Untitled_v4 (Autodesk Fusion 360 design; units mm, degrees)
Autodesk Fusion 360 part; units mm, degrees
(part 1 of 11)
sketch "Sketch1" plane through (0, 0, 0) normal (0, 1, 0) x (1, 0, 0)
  line L0 (0, -20) -> (0, 0)
  line L1 (0, 0) -> (20, 0)
  line L2 (20, 0) -> (0, -20)
  constraint coincident L0.end L1.start
  constraint vertical L0
  constraint perpendicular L0 L1
extrude "Extrude1" add sketch "Sketch1" along normal blind 220
extrude "Extrude2" add 1 faces at (6.6667, 73.3333, 0) along direction (0, 0, -1) blind 3
extrude "Extrude3" add 1 faces at (0, 73.3333, 12.3333) along direction (-1, 0, 0) blind 3
sketch "Sketch2" plane through (0, 0, -3) normal (0, 0, -1) x (1, 0, 0)
  line L0 (20, 0) -> (-3, 0)
  line L1 (-3, 0) -> (-3, -220)
  line L2 (-3, -220) -> (20, -220)
  line L3 (20, -220) -> (20, 0)
  line L4 (19.7694, -145.5685) -> (19.7946, -145.5378)
  line L5 (19.7422, -145.5975) -> (19.7694, -145.5685)
  line L6 (19.8738, -145.4005) -> (19.8878, -145.3633)
  line L7 (19.8177, -145.5055) -> (19.8387, -145.4717)
  line L8 (19.8878, -145.3633) -> (19.8993, -145.3253)
  line L9 (19.7946, -145.5378) -> (19.8177, -145.5055)
  line L10 (19.8574, -145.4367) -> (19.8738, -145.4005)
  line L11 (19.9083, -145.2866) -> (19.9148, -145.2474)
  line L12 (19.8574, -145.4367) -> (19.8738, -145.4005)
  line L13 (19.7946, -145.5378) -> (19.8177, -145.5055)
  line L14 (19.7422, -145.5975) -> (19.7694, -145.5685)
  line L15 (19.8738, -145.4005) -> (19.8878, -145.3633)
  arc A0 (19.92, -140.4997) -> (19.42, -139.9997) centre (19.42, -140.4997) ccw
  arc A1 (19.92, -140.4997) -> (19.42, -139.9997) centre (19.42, -140.4997) ccw
  line L16 (18.42, -139.9997) -> (19.42, -139.9997)
  line L17 (14.7514, -139.9997) -> (14.7117, -140.001)
  line L18 (14.7117, -139.9984) -> (14.7514, -139.9997)
  line L19 (14.7117, -139.9984) -> (14.7514, -139.9997)
  line L20 (14.7514, -139.9997) -> (14.7117, -140.001)
  arc A2 (19.42, -139.9997) -> (19.92, -139.4997) centre (19.42, -139.4997) ccw
  line L21 (18.42, -139.9997) -> (14.7514, -139.9997)
  line L22 (19.8993, -145.3253) -> (19.9083, -145.2866)
  line L23 (18.42, -139.9997) -> (14.7514, -139.9997)
  line L24 (18.42, -139.9997) -> (19.42, -139.9997)
  arc A3 (19.42, -139.9997) -> (19.92, -139.4997) centre (19.42, -139.4997) ccw
  line L25 (14.7514, -139.9997) -> (18.42, -139.9997)
  line L26 (14.7514, -139.9997) -> (18.42, -139.9997)
  line L27 (19.42, -139.9997) -> (18.42, -139.9997)
  line L28 (19.42, -139.9997) -> (18.42, -139.9997)
  line L29 (14.3819, -139.8742) -> (14.4142, -139.8974)
  line L30 (14.3222, -139.8219) -> (14.3512, -139.849)
  line L31 (14.5191, -140.0459) -> (14.483, -140.0623)
  line L32 (14.4142, -140.102) -> (14.3819, -140.1251)
  line L33 (14.483, -140.0623) -> (14.4479, -140.081)
  line L34 (14.3222, -139.8219) -> (14.3512, -139.849)
  line L35 (14.4479, -139.9183) -> (14.483, -139.9371)
  line L36 (14.3512, -140.1503) -> (14.3222, -140.1775)
  line L37 (14.3512, -139.849) -> (14.3819, -139.8742)
  line L38 (9.92, -146.3044) -> (9.7152, -146.0997)
  line L39 (14.483, -140.0623) -> (14.4479, -140.081)
  line L40 (14.3819, -139.8742) -> (14.4142, -139.8974)
  line L41 (14.483, -139.9371) -> (14.5191, -139.9534)
  line L42 (12.7593, -146.0997) -> (10.127, -146.0997)
  line L43 (14.3512, -139.849) -> (14.3819, -139.8742)
  line L44 (14.3819, -140.1251) -> (14.3512, -140.1503)
  line L45 (14.4142, -139.8974) -> (14.4479, -139.9183)
  line L46 (14.4479, -140.081) -> (14.4142, -140.102)
  line L47 (14.4479, -140.081) -> (14.4142, -140.102)
  line L48 (14.483, -139.9371) -> (14.5191, -139.9534)
  line L49 (14.3819, -140.1251) -> (14.3512, -140.1503)
  line L50 (14.4142, -139.8974) -> (14.4479, -139.9183)
  line L51 (14.4479, -139.9183) -> (14.483, -139.9371)
  line L52 (14.3512, -140.1503) -> (14.3222, -140.1775)
  line L53 (14.5191, -140.0459) -> (14.483, -140.0623)
  line L54 (14.4142, -140.102) -> (14.3819, -140.1251)
  line L55 (14.5943, -140.0203) -> (14.5563, -140.0319)
  line L56 (14.6722, -139.9945) -> (14.7117, -139.9984)
  line L57 (14.633, -139.988) -> (14.6722, -139.9945)
  line L58 (14.5943, -140.0203) -> (14.5563, -140.0319)
  line L59 (14.5563, -139.9674) -> (14.5943, -139.979)
  line L60 (14.6722, -140.0049) -> (14.633, -140.0113)
  line L61 (14.633, -140.0113) -> (14.5943, -140.0203)
  line L62 (14.6722, -139.9945) -> (14.7117, -139.9984)
  line L63 (14.633, -139.988) -> (14.6722, -139.9945)
  line L64 (14.6722, -140.0049) -> (14.633, -140.0113)
  line L65 (14.7117, -140.001) -> (14.6722, -140.0049)
  line L66 (14.5943, -139.979) -> (14.633, -139.988)
  line L67 (14.7117, -140.001) -> (14.6722, -140.0049)
  line L68 (14.5943, -139.979) -> (14.633, -139.988)
  line L69 (14.633, -140.0113) -> (14.5943, -140.0203)
  line L70 (14.5563, -139.9674) -> (14.5943, -139.979)
  line L71 (14.5563, -140.0319) -> (14.5191, -140.0459)
  line L72 (14.5191, -139.9534) -> (14.5563, -139.9674)
  line L73 (14.5563, -140.0319) -> (14.5191, -140.0459)
  line L74 (14.5191, -139.9534) -> (14.5563, -139.9674)
  line L75 (10.127, -146.0997) -> (9.92, -146.3044)
  line L76 (7.0807, -146.0997) -> (4.42, -143.439)
  line L77 (1.72, -144.4997) -> (3.3593, -144.4997)
  arc A4 (13.0414, -141.4582) -> (13.1828, -141.7997) centre (13.1828, -141.5997) ccw
  arc A5 (6.6572, -141.7997) -> (6.7986, -141.4582) centre (6.6572, -141.5997) ccw
  line L78 (9.92, -146.3044) -> (9.7152, -146.0997)
  line L79 (6.7986, -141.4582) -> (5.5178, -140.1775)
  line L80 (0.0978, -145.5975) -> (1.3786, -146.8782)
  line L81 (-0.08, -140.4997) -> (-0.08, -141.4997)
  line L82 (4.42, -143.439) -> (4.42, -141.7997)
  line L83 (4.42, -143.439) -> (4.42, -141.7997)
  line L84 (0.0978, -145.5975) -> (1.3786, -146.8782)
  line L85 (1.72, -144.4997) -> (3.3593, -144.4997)
  arc A6 (6.6572, -141.7997) -> (6.7986, -141.4582) centre (6.6572, -141.5997) ccw
  line L86 (7.0807, -146.0997) -> (4.42, -143.439)
  line L87 (4.42, -141.7997) -> (6.6572, -141.7997)
  line L88 (4.42, -141.7997) -> (6.6572, -141.7997)
  line L89 (-0.08, -140.4997) -> (-0.08, -141.4997)
  line L90 (6.7986, -141.4582) -> (5.5178, -140.1775)
  arc A7 (13.0414, -141.4582) -> (13.1828, -141.7997) centre (13.1828, -141.5997) ccw
  line L91 (12.7593, -146.0997) -> (10.127, -146.0997)
  line L92 (10.127, -146.0997) -> (9.92, -146.3044)
  line L93 (5.3209, -140.0459) -> (5.2837, -140.0319)
  line L94 (5.3209, -139.9534) -> (5.357, -139.9371)
  line L95 (5.357, -139.9371) -> (5.3921, -139.9183)
  line L96 (5.2837, -139.9674) -> (5.3209, -139.9534)
  line L97 (5.3209, -140.0459) -> (5.2837, -140.0319)
  line L98 (5.4888, -139.849) -> (5.5178, -139.8219)
  line L99 (5.4258, -140.102) -> (5.3921, -140.081)
  line L100 (5.0886, -139.9997) -> (5.1283, -139.9984)
  line L101 (5.3921, -140.081) -> (5.357, -140.0623)
  line L102 (5.3209, -139.9534) -> (5.357, -139.9371)
  line L103 (5.1283, -140.001) -> (5.0886, -139.9997)
  line L104 (5.0886, -139.9997) -> (5.1283, -139.9984)
  line L105 (5.1283, -140.001) -> (5.0886, -139.9997)
  line L106 (5.4581, -140.1251) -> (5.4258, -140.102)
  line L107 (5.4258, -139.8974) -> (5.4581, -139.8742)
  line L108 (5.2837, -139.9674) -> (5.3209, -139.9534)
  line L109 (5.3921, -139.9183) -> (5.4258, -139.8974)
  line L110 (5.357, -139.9371) -> (5.3921, -139.9183)
  line L111 (5.357, -140.0623) -> (5.3209, -140.0459)
  line L112 (5.4888, -140.1503) -> (5.4581, -140.1251)
  line L113 (5.3921, -139.9183) -> (5.4258, -139.8974)
  line L114 (5.4581, -140.1251) -> (5.4258, -140.102)
  line L115 (5.4258, -140.102) -> (5.3921, -140.081)
  line L116 (5.4258, -139.8974) -> (5.4581, -139.8742)
  line L117 (5.4581, -139.8742) -> (5.4888, -139.849)
  line L118 (5.3921, -140.081) -> (5.357, -140.0623)
  line L119 (5.357, -140.0623) -> (5.3209, -140.0459)
  line L120 (5.5178, -140.1775) -> (5.4888, -140.1503)
  line L121 (5.5178, -140.1775) -> (5.4888, -140.1503)
  line L122 (5.4888, -139.849) -> (5.5178, -139.8219)
  line L123 (-0.0174, -145.4367) -> (0.0013, -145.4717)
  line L124 (-0.0593, -145.3253) -> (-0.0478, -145.3633)
  line L125 (0.0706, -145.5685) -> (0.0978, -145.5975)
  line L126 (0.0454, -145.5378) -> (0.0706, -145.5685)
  line L127 (0.0454, -145.5378) -> (0.0706, -145.5685)
  line L128 (-0.0174, -145.4367) -> (0.0013, -145.4717)
  line L129 (-0.08, -141.4997) -> (-0.08, -145.0997)
  line L130 (-0.0683, -145.2866) -> (-0.0593, -145.3253)
  line L131 (-0.0593, -145.3253) -> (-0.0478, -145.3633)
  line L132 (-0.08, -145.0997) -> (-0.0787, -145.2079)
  line L133 (-0.0748, -145.2474) -> (-0.0683, -145.2866)
  line L134 (-0.0338, -145.4005) -> (-0.0174, -145.4367)
  line L135 (-0.0338, -145.4005) -> (-0.0174, -145.4367)
  line L136 (-0.0787, -145.2079) -> (-0.0748, -145.2474)
  line L137 (-0.0478, -145.3633) -> (-0.0338, -145.4005)
  line L138 (-0.08, -141.4997) -> (-0.08, -145.0997)
  line L139 (1.72, -146.7368) -> (1.72, -144.4997)
  line L140 (1.72, -146.7368) -> (1.72, -144.4997)
  line L141 (-0.0748, -145.2474) -> (-0.0683, -145.2866)
  line L142 (0.0706, -145.5685) -> (0.0978, -145.5975)
  line L143 (-0.0787, -145.2079) -> (-0.0748, -145.2474)
  line L144 (0.0223, -145.5055) -> (0.0454, -145.5378)
  line L145 (0.0013, -145.4717) -> (0.0223, -145.5055)
  line L146 (-0.08, -145.0997) -> (-0.0787, -145.2079)
  line L147 (0.0013, -145.4717) -> (0.0223, -145.5055)
  line L148 (-0.0478, -145.3633) -> (-0.0338, -145.4005)
  line L149 (0.0223, -145.5055) -> (0.0454, -145.5378)
  line L150 (-0.0683, -145.2866) -> (-0.0593, -145.3253)
  line L151 (18.12, -144.4997) -> (18.12, -146.7368)
  line L152 (16.4807, -144.4997) -> (18.12, -144.4997)
  line L153 (15.42, -141.7997) -> (15.42, -143.439)
  line L154 (15.42, -141.7997) -> (15.42, -143.439)
  line L155 (16.4807, -144.4997) -> (18.12, -144.4997)
  line L156 (18.12, -144.4997) -> (18.12, -146.7368)
  line L157 (5.207, -139.988) -> (5.2457, -139.979)
  line L158 (5.1283, -139.9984) -> (5.1678, -139.9945)
  line L159 (5.2457, -140.0203) -> (5.207, -140.0113)
  line L160 (5.1283, -139.9984) -> (5.1678, -139.9945)
  line L161 (5.2457, -139.979) -> (5.2837, -139.9674)
  line L162 (5.1678, -140.0049) -> (5.1283, -140.001)
  line L163 (5.2457, -140.0203) -> (5.207, -140.0113)
  line L164 (5.1678, -139.9945) -> (5.207, -139.988)
  line L165 (5.1678, -139.9945) -> (5.207, -139.988)
  line L166 (5.207, -140.0113) -> (5.1678, -140.0049)
  line L167 (5.207, -140.0113) -> (5.1678, -140.0049)
  line L168 (5.1678, -140.0049) -> (5.1283, -140.001)
  line L169 (5.207, -139.988) -> (5.2457, -139.979)
  line L170 (5.2837, -140.0319) -> (5.2457, -140.0203)
  line L171 (5.4581, -139.8742) -> (5.4888, -139.849)
  line L172 (5.4888, -140.1503) -> (5.4581, -140.1251)
  line L173 (5.2837, -140.0319) -> (5.2457, -140.0203)
  arc A8 (0.42, -139.9997) -> (-0.08, -140.4997) centre (0.42, -140.4997) ccw
  arc A9 (-0.08, -139.4997) -> (0.42, -139.9997) centre (0.42, -139.4997) ccw
  arc A10 (0.42, -139.9997) -> (-0.08, -140.4997) centre (0.42, -140.4997) ccw
  line L174 (1.42, -139.9997) -> (0.42, -139.9997)
  line L175 (5.0886, -139.9997) -> (1.42, -139.9997)
  line L176 (1.42, -139.9997) -> (5.0886, -139.9997)
  line L177 (0.42, -139.9997) -> (1.42, -139.9997)
  arc A11 (-0.08, -139.4997) -> (0.42, -139.9997) centre (0.42, -139.4997) ccw
  line L178 (0.42, -139.9997) -> (1.42, -139.9997)
  line L179 (1.42, -139.9997) -> (5.0886, -139.9997)
  line L180 (1.42, -139.9997) -> (0.42, -139.9997)
  line L181 (5.0886, -139.9997) -> (1.42, -139.9997)
  line L182 (5.2457, -139.979) -> (5.2837, -139.9674)
  line L183 (3.6807, -162.6997) -> (1.72, -162.6997)
  line L184 (7.0807, -166.0997) -> (3.6807, -162.6997)
  line L185 (0.0978, -165.5975) -> (1.3786, -166.8782)
  line L186 (3.6807, -162.6997) -> (1.72, -162.6997)
  line L187 (3.3593, -164.4997) -> (6.02, -167.1603)
  arc A12 (1.3786, -166.8782) -> (1.72, -166.7368) centre (1.52, -166.7368) ccw
  line L188 (1.72, -164.4997) -> (3.3593, -164.4997)
  arc A13 (1.3786, -166.8782) -> (1.72, -166.7368) centre (1.52, -166.7368) ccw
  line L189 (7.0807, -166.0997) -> (3.6807, -162.6997)
  line L190 (0.0978, -165.5975) -> (1.3786, -166.8782)
  line L191 (3.3593, -164.4997) -> (6.02, -167.1603)
  line L192 (1.72, -166.7368) -> (1.72, -164.4997)
  line L193 (1.72, -166.7368) -> (1.72, -164.4997)
  line L194 (1.72, -175.4997) -> (1.72, -173.2625)
  line L195 (-0.0593, -174.674) -> (-0.0683, -174.7127)
  line L196 (-0.0338, -174.5988) -> (-0.0478, -174.636)
  arc A14 (1.72, -173.2625) -> (1.3786, -173.1211) centre (1.52, -173.2625) ccw
  line L197 (0.0454, -174.4616) -> (0.0223, -174.4938)
  line L198 (-0.0174, -174.5626) -> (-0.0338, -174.5988)
  line L199 (0.0706, -174.4308) -> (0.0454, -174.4616)
  line L200 (1.72, -175.4997) -> (1.72, -173.2625)
  line L201 (0.0013, -174.5276) -> (-0.0174, -174.5626)
  line L202 (-0.0683, -174.7127) -> (-0.0748, -174.7519)
  line L203 (1.3786, -173.1211) -> (0.0978, -174.4019)
  line L204 (-0.0787, -174.7914) -> (-0.08, -174.8997)
  line L205 (0.0223, -174.4938) -> (0.0013, -174.5276)
  line L206 (-0.0787, -174.7914) -> (-0.08, -174.8997)
  line L207 (0.0454, -174.4616) -> (0.0223, -174.4938)
  line L208 (0.0013, -174.5276) -> (-0.0174, -174.5626)
  line L209 (-0.0748, -174.7519) -> (-0.0787, -174.7914)
  line L210 (0.0223, -174.4938) -> (0.0013, -174.5276)
  arc A15 (1.72, -173.2625) -> (1.3786, -173.1211) centre (1.52, -173.2625) ccw
  line L211 (-0.0683, -174.7127) -> (-0.0748, -174.7519)
  line L212 (0.0978, -174.4019) -> (0.0706, -174.4308)
  line L213 (0.0706, -174.4308) -> (0.0454, -174.4616)
  line L214 (0.0978, -174.4019) -> (0.0706, -174.4308)
  line L215 (-0.0174, -174.5626) -> (-0.0338, -174.5988)
  line L216 (1.3786, -173.1211) -> (0.0978, -174.4019)
  line L217 (-0.0748, -174.7519) -> (-0.0787, -174.7914)
  line L218 (-0.0338, -174.5988) -> (-0.0478, -174.636)
  line L219 (-0.0478, -174.636) -> (-0.0593, -174.674)
  line L220 (-0.0593, -174.674) -> (-0.0683, -174.7127)
  line L221 (-0.0478, -174.636) -> (-0.0593, -174.674)
  circle A16 centre (9.92, -109.9997) radius 2.1
  line L222 (6.02, -110.1995) -> (6.02, -112.839)
  line L223 (13.82, -112.839) -> (13.82, -110.1995)
  circle A17 centre (9.92, -109.9997) radius 2.1
  line L224 (-0.0174, -165.4367) -> (0.0013, -165.4717)
  line L225 (1.72, -164.4997) -> (3.3593, -164.4997)
  line L226 (-0.0683, -165.2866) -> (-0.0593, -165.3253)
  line L227 (0.0454, -165.5378) -> (0.0706, -165.5685)
  line L228 (0.0706, -165.5685) -> (0.0978, -165.5975)
  line L229 (0.0013, -165.4717) -> (0.0223, -165.5055)
  line L230 (0.0223, -165.5055) -> (0.0454, -165.5378)
  line L231 (-0.0748, -165.2474) -> (-0.0683, -165.2866)
  line L232 (-0.0338, -165.4005) -> (-0.0174, -165.4367)
  line L233 (0.0454, -165.5378) -> (0.0706, -165.5685)
  line L234 (-0.0478, -165.3633) -> (-0.0338, -165.4005)
  line L235 (-0.0338, -165.4005) -> (-0.0174, -165.4367)
  line L236 (0.0223, -165.5055) -> (0.0454, -165.5378)
  line L237 (3.3593, -124.4997) -> (6.02, -127.1603)
  line L238 (13.82, -127.1603) -> (16.4807, -124.4997)
  line L239 (5.5178, -139.8219) -> (6.7986, -138.5411)
  line L240 (13.82, -127.1603) -> (16.4807, -124.4997)
  line L241 (3.3593, -124.4997) -> (6.02, -127.1603)
  line L242 (5.5178, -139.8219) -> (6.7986, -138.5411)
  line L243 (13.0414, -138.5411) -> (14.3222, -139.8219)
  arc A18 (1.3786, -126.8782) -> (1.72, -126.7368) centre (1.52, -126.7368) ccw
  arc A19 (18.12, -126.7368) -> (18.4614, -126.8782) centre (18.32, -126.7368) ccw
  line L244 (13.0414, -138.5411) -> (14.3222, -139.8219)
  line L245 (19.92, -139.4997) -> (19.92, -138.4997)
  arc A20 (18.12, -126.7368) -> (18.4614, -126.8782) centre (18.32, -126.7368) ccw
  line L246 (19.92, -139.4997) -> (19.92, -138.4997)
  arc A21 (1.3786, -126.8782) -> (1.72, -126.7368) centre (1.52, -126.7368) ccw
  line L247 (-0.08, -138.4997) -> (-0.08, -139.4997)
  line L248 (-0.08, -138.4997) -> (-0.08, -139.4997)
  line L249 (0.0706, -165.5685) -> (0.0978, -165.5975)
  line L250 (-0.0787, -165.2079) -> (-0.0748, -165.2474)
  line L251 (-0.0748, -165.2474) -> (-0.0683, -165.2866)
  line L252 (-0.0683, -165.2866) -> (-0.0593, -165.3253)
  line L253 (-0.0174, -165.4367) -> (0.0013, -165.4717)
  line L254 (-0.08, -165.0997) -> (-0.0787, -165.2079)
  line L255 (0.0013, -165.4717) -> (0.0223, -165.5055)
  line L256 (-0.0593, -165.3253) -> (-0.0478, -165.3633)
  line L257 (-0.08, -165.0997) -> (-0.0787, -165.2079)
  line L258 (-0.0787, -165.2079) -> (-0.0748, -165.2474)
  line L259 (-0.0478, -165.3633) -> (-0.0338, -165.4005)
  line L260 (-0.0593, -165.3253) -> (-0.0478, -165.3633)
  line L261 (6.02, -112.839) -> (3.3593, -115.4997)
  line L262 (-0.08, -114.8997) -> (-0.08, -125.0997)
  line L263 (1.72, -122.6997) -> (1.72, -117.2997)
  line L264 (10.127, -126.0997) -> (9.92, -126.3066)
  line L265 (12.7593, -126.0997) -> (10.127, -126.0997)
  line L266 (-0.08, -114.8997) -> (-0.08, -125.0997)
  line L267 (1.72, -122.6997) -> (1.72, -117.2997)
  line L268 (-0.0787, -114.7914) -> (-0.08, -114.8997)
  line L269 (1.72, -117.2997) -> (3.6807, -117.2997)
  line L270 (3.3593, -115.4997) -> (1.72, -115.4997)
  line L271 (-0.0683, -114.7127) -> (-0.0748, -114.7519)
  line L272 (-0.0478, -114.636) -> (-0.0593, -114.674)
  line L273 (0.0454, -114.4616) -> (0.0223, -114.4938)
  line L274 (-0.0748, -114.7519) -> (-0.0787, -114.7914)
  line L275 (0.0706, -114.4308) -> (0.0454, -114.4616)
  line L276 (1.72, -115.4997) -> (1.72, -113.2625)
  line L277 (-0.0338, -114.5988) -> (-0.0478, -114.636)
  line L278 (0.0223, -114.4938) -> (0.0013, -114.5276)
  line L279 (-0.0174, -114.5626) -> (-0.0338, -114.5988)
  line L280 (6.02, -112.839) -> (3.3593, -115.4997)
  line L281 (1.72, -115.4997) -> (1.72, -113.2625)
  line L282 (-0.0174, -114.5626) -> (-0.0338, -114.5988)
  line L283 (-0.0683, -114.7127) -> (-0.0748, -114.7519)
  line L284 (0.0978, -114.4019) -> (0.0706, -114.4308)
  line L285 (0.0013, -114.5276) -> (-0.0174, -114.5626)
  line L286 (-0.0593, -114.674) -> (-0.0683, -114.7127)
  line L287 (3.3593, -115.4997) -> (1.72, -115.4997)
  line L288 (0.0013, -114.5276) -> (-0.0174, -114.5626)
  line L289 (0.0978, -114.4019) -> (0.0706, -114.4308)
  line L290 (1.3786, -113.1211) -> (0.0978, -114.4019)
  line L291 (-0.0787, -114.7914) -> (-0.08, -114.8997)
  line L292 (0.0706, -114.4308) -> (0.0454, -114.4616)
  line L293 (1.72, -117.2997) -> (3.6807, -117.2997)
  line L294 (-0.0338, -114.5988) -> (-0.0478, -114.636)
  arc A22 (1.72, -113.2625) -> (1.3786, -113.1211) centre (1.52, -113.2625) ccw
  line L295 (-0.0478, -114.636) -> (-0.0593, -114.674)
  line L296 (0.0454, -114.4616) -> (0.0223, -114.4938)
  arc A23 (1.72, -113.2625) -> (1.3786, -113.1211) centre (1.52, -113.2625) ccw
  line L297 (1.3786, -113.1211) -> (0.0978, -114.4019)
  line L298 (-0.0748, -114.7519) -> (-0.0787, -114.7914)
  line L299 (-0.0593, -114.674) -> (-0.0683, -114.7127)
  line L300 (0.0223, -114.4938) -> (0.0013, -114.5276)
  line L301 (0.0223, -134.4938) -> (0.0013, -134.5276)
  line L302 (0.0013, -134.5276) -> (-0.0174, -134.5626)
  line L303 (-0.0683, -134.7127) -> (-0.0748, -134.7519)
  line L304 (-0.08, -134.8997) -> (-0.08, -138.4997)
  line L305 (0.0978, -134.4019) -> (0.0706, -134.4308)
  line L306 (-0.0338, -134.5988) -> (-0.0478, -134.636)
  line L307 (0.0223, -134.4938) -> (0.0013, -134.5276)
  line L308 (0.0013, -134.5276) -> (-0.0174, -134.5626)
  line L309 (-0.0748, -134.7519) -> (-0.0787, -134.7914)
  line L310 (-0.0478, -134.636) -> (-0.0593, -134.674)
  line L311 (0.0978, -134.4019) -> (0.0706, -134.4308)
  line L312 (-0.0174, -134.5626) -> (-0.0338, -134.5988)
  line L313 (-0.0787, -134.7914) -> (-0.08, -134.8997)
  line L314 (0.0706, -134.4308) -> (0.0454, -134.4616)
  line L315 (6.6572, -138.1997) -> (4.42, -138.1997)
  line L316 (6.02, -129.7998) -> (6.2199, -129.9997)
  arc A24 (6.7986, -138.5411) -> (6.6572, -138.1997) centre (6.6572, -138.3997) ccw
  line L317 (4.42, -138.1997) -> (4.42, -136.5603)
  line L318 (6.02, -129.7998) -> (6.2199, -129.9997)
  arc A25 (6.7986, -138.5411) -> (6.6572, -138.1997) centre (6.6572, -138.3997) ccw
  line L319 (3.3593, -135.4997) -> (1.72, -135.4997)
  line L320 (3.3593, -135.4997) -> (1.72, -135.4997)
  line L321 (4.42, -138.1997) -> (4.42, -136.5603)
  line L322 (6.6572, -138.1997) -> (4.42, -138.1997)
  line L323 (6.02, -130.1995) -> (6.02, -132.839)
  arc A26 (1.72, -133.2625) -> (1.3786, -133.1211) centre (1.52, -133.2625) ccw
  line L324 (4.42, -136.5603) -> (7.0807, -133.8997)
  line L325 (6.02, -127.1603) -> (6.02, -129.7998)
  line L326 (6.2199, -129.9997) -> (6.02, -130.1995)
  line L327 (6.02, -132.839) -> (3.3593, -135.4997)
  line L328 (1.3786, -133.1211) -> (0.0978, -134.4019)
  line L329 (1.3786, -133.1211) -> (0.0978, -134.4019)
  line L330 (1.72, -135.4997) -> (1.72, -133.2625)
  arc A27 (1.72, -133.2625) -> (1.3786, -133.1211) centre (1.52, -133.2625) ccw
  line L331 (4.42, -136.5603) -> (7.0807, -133.8997)
  line L332 (6.02, -127.1603) -> (6.02, -129.7998)
  line L333 (6.2199, -129.9997) -> (6.02, -130.1995)
  line L334 (6.02, -130.1995) -> (6.02, -132.839)
  line L335 (6.02, -132.839) -> (3.3593, -135.4997)
  line L336 (1.72, -135.4997) -> (1.72, -133.2625)
  line L337 (13.6201, -129.9997) -> (13.82, -129.7998)
  line L338 (13.82, -132.839) -> (13.82, -130.1995)
  line L339 (9.92, -133.6949) -> (10.127, -133.8997)
  arc A28 (13.1828, -138.1997) -> (13.0414, -138.5411) centre (13.1828, -138.3997) ccw
  line L340 (9.7152, -133.8997) -> (9.92, -133.6949)
  line L341 (13.82, -129.7998) -> (13.82, -127.1603)
  line L342 (15.42, -136.5603) -> (15.42, -138.1997)
  line L343 (13.82, -129.7998) -> (13.82, -127.1603)
  line L344 (13.82, -130.1995) -> (13.6201, -129.9997)
  line L345 (19.7946, -134.4616) -> (19.7694, -134.4308)
  line L346 (19.92, -138.4997) -> (19.92, -134.8311)
  line L347 (16.4807, -135.4997) -> (13.82, -132.839)
  line L348 (18.12, -135.4997) -> (16.4807, -135.4997)
  circle A29 centre (9.92, -129.9997) radius 2.1
  circle A30 centre (9.92, -129.9997) radius 2.1
  line L349 (7.0807, -133.8997) -> (9.7152, -133.8997)
  line L350 (16.4807, -135.4997) -> (13.82, -132.839)
  line L351 (7.0807, -133.8997) -> (9.7152, -133.8997)
  line L352 (19.8878, -134.636) -> (19.8738, -134.5988)
  line L353 (-0.0174, -125.4367) -> (0.0013, -125.4717)
  line L354 (1.72, -124.4997) -> (3.3593, -124.4997)
  line L355 (0.0013, -125.4717) -> (0.0223, -125.5055)
  line L356 (-0.0683, -125.2866) -> (-0.0593, -125.3253)
  line L357 (-0.08, -125.0997) -> (-0.0787, -125.2079)
  line L358 (0.0706, -125.5685) -> (0.0978, -125.5975)
  line L359 (-0.08, -125.0997) -> (-0.0787, -125.2079)
  line L360 (-0.0478, -125.3633) -> (-0.0338, -125.4005)
  line L361 (-0.0338, -125.4005) -> (-0.0174, -125.4367)
  line L362 (-0.0593, -125.3253) -> (-0.0478, -125.3633)
  line L363 (1.72, -124.4997) -> (3.3593, -124.4997)
  line L364 (-0.0338, -125.4005) -> (-0.0174, -125.4367)
  line L365 (0.0223, -125.5055) -> (0.0454, -125.5378)
  line L366 (-0.0478, -125.3633) -> (-0.0338, -125.4005)
  line L367 (-0.0593, -125.3253) -> (-0.0478, -125.3633)
  line L368 (0.0978, -125.5975) -> (1.3786, -126.8782)
  line L369 (-0.0748, -125.2474) -> (-0.0683, -125.2866)
  line L370 (-0.0748, -125.2474) -> (-0.0683, -125.2866)
  line L371 (-0.0683, -125.2866) -> (-0.0593, -125.3253)
  line L372 (0.0454, -125.5378) -> (0.0706, -125.5685)
  line L373 (0.0223, -125.5055) -> (0.0454, -125.5378)
  line L374 (1.72, -126.7368) -> (1.72, -124.4997)
  line L375 (1.72, -126.7368) -> (1.72, -124.4997)
  line L376 (0.0706, -125.5685) -> (0.0978, -125.5975)
  line L377 (0.0013, -125.4717) -> (0.0223, -125.5055)
  line L378 (3.6807, -122.6997) -> (1.72, -122.6997)
  line L379 (-0.0787, -125.2079) -> (-0.0748, -125.2474)
  line L380 (-0.0174, -125.4367) -> (0.0013, -125.4717)
  line L381 (3.6807, -122.6997) -> (1.72, -122.6997)
  line L382 (0.0978, -125.5975) -> (1.3786, -126.8782)
  line L383 (0.0454, -125.5378) -> (0.0706, -125.5685)
  line L384 (-0.0787, -125.2079) -> (-0.0748, -125.2474)
  line L385 (19.8574, -134.5626) -> (19.8387, -134.5276)
  line L386 (19.9187, -134.7914) -> (19.9148, -134.7519)
  line L387 (19.7422, -134.4019) -> (18.4614, -133.1211)
  line L388 (19.8878, -134.636) -> (19.8738, -134.5988)
  line L389 (19.8574, -134.5626) -> (19.8387, -134.5276)
  line L390 (19.9083, -134.7127) -> (19.8993, -134.674)
  line L391 (19.92, -138.4997) -> (19.92, -134.8311)
  line L392 (19.8387, -134.5276) -> (19.8177, -134.4938)
  line L393 (19.9148, -134.7519) -> (19.9083, -134.7127)
  line L394 (19.8177, -134.4938) -> (19.7946, -134.4616)
  line L395 (19.8993, -134.674) -> (19.8878, -134.636)
  line L396 (19.9148, -134.7519) -> (19.9083, -134.7127)
  line L397 (19.7946, -134.4616) -> (19.7694, -134.4308)
  line L398 (19.7694, -134.4308) -> (19.7422, -134.4019)
  line L399 (19.8177, -134.4938) -> (19.7946, -134.4616)
  line L400 (19.9187, -134.7914) -> (19.9148, -134.7519)
  line L401 (12.7593, -133.8997) -> (15.42, -136.5603)
  line L402 (15.42, -138.1997) -> (13.1828, -138.1997)
  line L403 (13.6201, -129.9997) -> (13.82, -129.7998)
  line L404 (10.127, -133.8997) -> (12.7593, -133.8997)
  line L405 (13.82, -130.1995) -> (13.6201, -129.9997)
  line L406 (15.42, -136.5603) -> (15.42, -138.1997)
  line L407 (13.82, -132.839) -> (13.82, -130.1995)
  line L408 (10.127, -133.8997) -> (12.7593, -133.8997)
  line L409 (9.92, -133.6949) -> (10.127, -133.8997)
  line L410 (12.7593, -133.8997) -> (15.42, -136.5603)
  line L411 (15.42, -138.1997) -> (13.1828, -138.1997)
  line L412 (9.7152, -133.8997) -> (9.92, -133.6949)
  arc A31 (13.1828, -138.1997) -> (13.0414, -138.5411) centre (13.1828, -138.3997) ccw
  line L413 (19.8387, -134.5276) -> (19.8177, -134.4938)
  line L414 (18.12, -133.2625) -> (18.12, -135.4997)
  line L415 (18.12, -133.2625) -> (18.12, -135.4997)
  line L416 (19.7694, -134.4308) -> (19.7422, -134.4019)
  arc A32 (18.4614, -133.1211) -> (18.12, -133.2625) centre (18.32, -133.2625) ccw
  line L417 (18.12, -135.4997) -> (16.4807, -135.4997)
  line L418 (19.8738, -134.5988) -> (19.8574, -134.5626)
  line L419 (19.8993, -134.674) -> (19.8878, -134.636)
  line L420 (19.92, -134.8311) -> (19.9187, -134.7914)
  line L421 (19.7422, -134.4019) -> (18.4614, -133.1211)
  arc A33 (18.4614, -133.1211) -> (18.12, -133.2625) centre (18.32, -133.2625) ccw
  line L422 (19.9083, -134.7127) -> (19.8993, -134.674)
  line L423 (19.92, -134.8311) -> (19.9187, -134.7914)
  line L424 (19.8738, -134.5988) -> (19.8574, -134.5626)
  line L425 (19.92, -125.0997) -> (19.92, -114.8997)
  line L426 (16.1593, -122.6997) -> (12.7593, -126.0997)
  line L427 (3.6807, -117.2997) -> (7.0807, -113.8997)
  line L428 (19.92, -125.0997) -> (19.92, -114.8997)
  line L429 (19.8993, -114.674) -> (19.8878, -114.636)
  line L430 (18.12, -113.2625) -> (18.12, -115.4997)
  line L431 (16.1593, -122.6997) -> (12.7593, -126.0997)
  line L432 (19.8177, -114.4938) -> (19.7946, -114.4616)
  line L433 (16.4807, -115.4997) -> (13.82, -112.839)
  line L434 (18.12, -115.4997) -> (16.4807, -115.4997)
  line L435 (16.4807, -115.4997) -> (13.82, -112.839)
  line L436 (12.7593, -113.8997) -> (16.1593, -117.2997)
  line L437 (7.0807, -126.0997) -> (3.6807, -122.6997)
  line L438 (12.7593, -113.8997) -> (16.1593, -117.2997)
  line L439 (7.0807, -126.0997) -> (3.6807, -122.6997)
  line L440 (3.6807, -117.2997) -> (7.0807, -113.8997)
  line L441 (19.8993, -114.674) -> (19.8878, -114.636)
  line L442 (19.9083, -114.7127) -> (19.8993, -114.674)
  line L443 (19.8878, -114.636) -> (19.8738, -114.5988)
  arc A34 (18.4614, -113.1211) -> (18.12, -113.2625) centre (18.32, -113.2625) ccw
  line L444 (18.12, -122.6997) -> (16.1593, -122.6997)
  line L445 (19.8738, -114.5988) -> (19.8574, -114.5626)
  line L446 (19.8738, -114.5988) -> (19.8574, -114.5626)
  line L447 (19.7422, -114.4019) -> (18.4614, -113.1211)
  line L448 (18.12, -122.6997) -> (16.1593, -122.6997)
  line L449 (16.1593, -117.2997) -> (18.12, -117.2997)
  line L450 (19.7694, -114.4308) -> (19.7422, -114.4019)
  line L451 (19.92, -114.8997) -> (19.9187, -114.7914)
  line L452 (19.8387, -114.5276) -> (19.8177, -114.4938)
  line L453 (19.92, -114.8997) -> (19.9187, -114.7914)
  line L454 (19.9083, -114.7127) -> (19.8993, -114.674)
  line L455 (19.7946, -114.4616) -> (19.7694, -114.4308)
  line L456 (19.7422, -114.4019) -> (18.4614, -113.1211)
  line L457 (19.8878, -114.636) -> (19.8738, -114.5988)
  line L458 (18.12, -117.2997) -> (18.12, -122.6997)
  line L459 (19.9148, -114.7519) -> (19.9083, -114.7127)
  line L460 (19.8177, -114.4938) -> (19.7946, -114.4616)
  line L461 (16.1593, -117.2997) -> (18.12, -117.2997)
  line L462 (19.9187, -114.7914) -> (19.9148, -114.7519)
  line L463 (19.8574, -114.5626) -> (19.8387, -114.5276)
  line L464 (19.7946, -114.4616) -> (19.7694, -114.4308)
  line L465 (18.12, -117.2997) -> (18.12, -122.6997)
  line L466 (18.12, -115.4997) -> (16.4807, -115.4997)
  arc A35 (18.4614, -113.1211) -> (18.12, -113.2625) centre (18.32, -113.2625) ccw
  line L467 (19.9148, -114.7519) -> (19.9083, -114.7127)
  line L468 (19.7694, -114.4308) -> (19.7422, -114.4019)
  line L469 (19.9187, -114.7914) -> (19.9148, -114.7519)
  line L470 (19.8574, -114.5626) -> (19.8387, -114.5276)
  line L471 (19.8387, -114.5276) -> (19.8177, -114.4938)
  line L472 (18.12, -113.2625) -> (18.12, -115.4997)
  line L473 (19.9187, -125.2079) -> (19.92, -125.0997)
  line L474 (19.8878, -125.3633) -> (19.8993, -125.3253)
  line L475 (16.4807, -124.4997) -> (18.12, -124.4997)
  line L476 (19.7946, -125.5378) -> (19.8177, -125.5055)
  line L477 (19.9083, -125.2866) -> (19.9148, -125.2474)
  line L478 (19.9187, -125.2079) -> (19.92, -125.0997)
  line L479 (19.8177, -125.5055) -> (19.8387, -125.4717)
  line L480 (19.9148, -125.2474) -> (19.9187, -125.2079)
  line L481 (19.8177, -125.5055) -> (19.8387, -125.4717)
  line L482 (19.7694, -125.5685) -> (19.7946, -125.5378)
  line L483 (12.7593, -126.0997) -> (10.127, -126.0997)
  line L484 (9.92, -126.3066) -> (9.713, -126.0997)
  line L485 (9.92, -113.6927) -> (10.127, -113.8997)
  line L486 (10.127, -126.0997) -> (9.92, -126.3066)
  line L487 (9.92, -113.6927) -> (10.127, -113.8997)
  line L488 (10.127, -113.8997) -> (12.7593, -113.8997)
  line L489 (7.0807, -113.8997) -> (9.713, -113.8997)
  line L490 (9.713, -126.0997) -> (7.0807, -126.0997)
  line L491 (9.713, -113.8997) -> (9.92, -113.6927)
  line L492 (7.0807, -113.8997) -> (9.713, -113.8997)
  line L493 (9.713, -126.0997) -> (7.0807, -126.0997)
  line L494 (9.92, -126.3066) -> (9.713, -126.0997)
  line L495 (9.713, -113.8997) -> (9.92, -113.6927)
  line L496 (10.127, -113.8997) -> (12.7593, -113.8997)
  line L497 (18.12, -124.4997) -> (18.12, -126.7368)
  line L498 (19.8993, -125.3253) -> (19.9083, -125.2866)
  line L499 (19.7946, -125.5378) -> (19.8177, -125.5055)
  line L500 (19.8574, -125.4367) -> (19.8738, -125.4005)
  line L501 (19.7694, -125.5685) -> (19.7946, -125.5378)
  line L502 (19.7422, -125.5975) -> (19.7694, -125.5685)
  line L503 (19.8738, -125.4005) -> (19.8878, -125.3633)
  line L504 (18.4614, -126.8782) -> (19.7422, -125.5975)
  line L505 (19.8738, -125.4005) -> (19.8878, -125.3633)
  line L506 (19.8387, -125.4717) -> (19.8574, -125.4367)
  line L507 (19.8993, -125.3253) -> (19.9083, -125.2866)
  line L508 (19.7422, -125.5975) -> (19.7694, -125.5685)
  line L509 (16.4807, -124.4997) -> (18.12, -124.4997)
  line L510 (19.8387, -125.4717) -> (19.8574, -125.4367)
  line L511 (19.8878, -125.3633) -> (19.8993, -125.3253)
  line L512 (19.8574, -125.4367) -> (19.8738, -125.4005)
  line L513 (19.9083, -125.2866) -> (19.9148, -125.2474)
  line L514 (18.12, -124.4997) -> (18.12, -126.7368)
  line L515 (19.9148, -125.2474) -> (19.9187, -125.2079)
  line L516 (18.4614, -126.8782) -> (19.7422, -125.5975)
  line L517 (18.12, -153.2625) -> (18.12, -155.4997)
  line L518 (19.9083, -154.7127) -> (19.8993, -154.674)
  line L519 (19.9148, -154.7519) -> (19.9083, -154.7127)
  line L520 (19.9187, -154.7914) -> (19.9148, -154.7519)
  line L521 (19.8574, -154.5626) -> (19.8387, -154.5276)
  line L522 (19.8738, -154.5988) -> (19.8574, -154.5626)
  line L523 (19.8387, -154.5276) -> (19.8177, -154.4938)
  line L524 (16.1593, -157.2997) -> (18.12, -157.2997)
  line L525 (19.8993, -154.674) -> (19.8878, -154.636)
  line L526 (18.12, -155.4997) -> (16.4807, -155.4997)
  line L527 (19.8878, -154.636) -> (19.8738, -154.5988)
  line L528 (19.7946, -154.4616) -> (19.7694, -154.4308)
  line L529 (16.1593, -157.2997) -> (18.12, -157.2997)
  line L530 (19.9187, -154.7914) -> (19.9148, -154.7519)
  line L531 (18.12, -155.4997) -> (16.4807, -155.4997)
  line L532 (19.7422, -154.4019) -> (18.4614, -153.1211)
  line L533 (12.7593, -153.8997) -> (16.1593, -157.2997)
  line L534 (12.7593, -153.8997) -> (16.1593, -157.2997)
  line L535 (19.92, -154.8997) -> (19.9187, -154.7914)
  line L536 (7.0807, -153.8997) -> (9.713, -153.8997)
  line L537 (19.92, -154.8997) -> (19.9187, -154.7914)
  line L538 (18.12, -153.2625) -> (18.12, -155.4997)
  line L539 (13.82, -147.1603) -> (16.4807, -144.4997)
  line L540 (7.0807, -153.8997) -> (9.713, -153.8997)
  arc A36 (1.3786, -146.8782) -> (1.72, -146.7368) centre (1.52, -146.7368) ccw
  line L541 (16.4807, -155.4997) -> (13.82, -152.839)
  line L542 (13.82, -147.1603) -> (16.4807, -144.4997)
  line L543 (16.4807, -155.4997) -> (13.82, -152.839)
  arc A37 (18.12, -146.7368) -> (18.4614, -146.8782) centre (18.32, -146.7368) ccw
  line L544 (3.3593, -144.4997) -> (6.02, -147.1603)
  arc A38 (18.12, -146.7368) -> (18.4614, -146.8782) centre (18.32, -146.7368) ccw
  arc A39 (1.3786, -146.8782) -> (1.72, -146.7368) centre (1.52, -146.7368) ccw
  line L545 (3.3593, -144.4997) -> (6.02, -147.1603)
  line L546 (-0.0338, -134.5988) -> (-0.0478, -134.636)
  line L547 (-0.0593, -134.674) -> (-0.0683, -134.7127)
  line L548 (-0.0787, -134.7914) -> (-0.08, -134.8997)
  line L549 (-0.0683, -134.7127) -> (-0.0748, -134.7519)
  line L550 (-0.0478, -134.636) -> (-0.0593, -134.674)
  line L551 (-0.0748, -134.7519) -> (-0.0787, -134.7914)
  line L552 (0.0706, -134.4308) -> (0.0454, -134.4616)
  line L553 (-0.0174, -134.5626) -> (-0.0338, -134.5988)
  line L554 (0.0454, -134.4616) -> (0.0223, -134.4938)
  line L555 (0.0454, -134.4616) -> (0.0223, -134.4938)
  line L556 (-0.0593, -134.674) -> (-0.0683, -134.7127)
  line L557 (-0.08, -134.8997) -> (-0.08, -138.4997)
  line L558 (0.0454, -94.4616) -> (0.0223, -94.4938)
  line L559 (0.0978, -94.4019) -> (0.0706, -94.4308)
  line L560 (19.8993, -194.674) -> (19.8878, -194.636)
  arc A40 (18.4614, -193.1211) -> (18.12, -193.2625) centre (18.32, -193.2625) ccw
  line L561 (19.7422, -194.4019) -> (18.4614, -193.1211)
  line L562 (-0.0683, -94.7127) -> (-0.0748, -94.7519)
  line L563 (-0.0478, -85.3633) -> (-0.0338, -85.4005)
  line L564 (19.92, -194.8997) -> (19.9187, -194.7914)
  line L565 (-0.0787, -94.7914) -> (-0.08, -94.8997)
  arc A41 (1.72, -93.2625) -> (1.3786, -93.1211) centre (1.52, -93.2625) ccw
  line L566 (-0.0174, -94.5626) -> (-0.0338, -94.5988)
  line L567 (19.8177, -194.4938) -> (19.7946, -194.4616)
  line L568 (18.12, -193.2625) -> (18.12, -195.4997)
  line L569 (19.8574, -194.5626) -> (19.8387, -194.5276)
  line L570 (1.72, -197.2997) -> (3.6807, -197.2997)
  line L571 (3.3593, -195.4997) -> (1.72, -195.4997)
  line L572 (3.3593, -195.4997) -> (1.72, -195.4997)
  arc A42 (1.72, -93.2625) -> (1.3786, -93.1211) centre (1.52, -93.2625) ccw
  line L573 (0.0013, -94.5276) -> (-0.0174, -94.5626)
  line L574 (19.8387, -194.5276) -> (19.8177, -194.4938)
  line L575 (19.8177, -194.4938) -> (19.7946, -194.4616)
  line L576 (19.9148, -194.7519) -> (19.9083, -194.7127)
  line L577 (19.8878, -194.636) -> (19.8738, -194.5988)
  line L578 (1.72, -95.4997) -> (1.72, -93.2625)
  line L579 (18.12, -195.4997) -> (16.4807, -195.4997)
  line L580 (19.7694, -194.4308) -> (19.7422, -194.4019)
  line L581 (-0.0748, -94.7519) -> (-0.0787, -94.7914)
  line L582 (-0.0787, -94.7914) -> (-0.08, -94.8997)
  line L583 (18.12, -195.4997) -> (16.4807, -195.4997)
  line L584 (16.4807, -195.4997) -> (13.82, -192.839)
  line L585 (0.0978, -94.4019) -> (0.0706, -94.4308)
  line L586 (-0.0174, -94.5626) -> (-0.0338, -94.5988)
  line L587 (-0.0338, -94.5988) -> (-0.0478, -94.636)
  arc A43 (18.4614, -193.1211) -> (18.12, -193.2625) centre (18.32, -193.2625) ccw
  line L588 (19.8387, -194.5276) -> (19.8177, -194.4938)
  line L589 (6.02, -89.7998) -> (6.2199, -89.9997)
  line L590 (0.0706, -94.4308) -> (0.0454, -94.4616)
  line L591 (6.2199, -89.9997) -> (6.02, -90.1995)
  line L592 (6.02, -92.839) -> (3.3593, -95.4997)
  line L593 (19.92, -194.8997) -> (19.9187, -194.7914)
  line L594 (6.02, -92.839) -> (3.3593, -95.4997)
  line L595 (19.7422, -194.4019) -> (18.4614, -193.1211)
  line L596 (6.02, -90.1995) -> (6.02, -92.839)
  line L597 (0.0454, -94.4616) -> (0.0223, -94.4938)
  line L598 (1.3786, -93.1211) -> (0.0978, -94.4019)
  line L599 (19.8878, -194.636) -> (19.8738, -194.5988)
  line L600 (-0.0593, -85.3253) -> (-0.0478, -85.3633)
  line L601 (-0.08, -85.0997) -> (-0.0787, -85.2079)
  line L602 (19.9187, -194.7914) -> (19.9148, -194.7519)
  line L603 (6.02, -47.1603) -> (6.02, -49.7998)
  line L604 (-0.0683, -94.7127) -> (-0.0748, -94.7519)
  line L605 (1.72, -95.4997) -> (1.72, -93.2625)
  line L606 (6.2199, -89.9997) -> (6.02, -90.1995)
  line L607 (16.4807, -195.4997) -> (13.82, -192.839)
  line L608 (6.02, -89.7998) -> (6.2199, -89.9997)
  line L609 (-0.0478, -94.636) -> (-0.0593, -94.674)
  line L610 (1.3786, -93.1211) -> (0.0978, -94.4019)
  line L611 (-0.0478, -94.636) -> (-0.0593, -94.674)
  line L612 (6.02, -90.1995) -> (6.02, -92.839)
  line L613 (19.9083, -194.7127) -> (19.8993, -194.674)
  line L614 (19.7946, -194.4616) -> (19.7694, -194.4308)
  line L615 (-0.0683, -85.2866) -> (-0.0593, -85.3253)
  line L616 (19.8993, -194.674) -> (19.8878, -194.636)
  line L617 (9.92, -46.3066) -> (9.713, -46.0997)
  line L618 (-0.08, -54.8997) -> (-0.08, -65.0997)
  line L619 (19.92, -65.0997) -> (19.92, -54.8997)
  line L620 (-0.08, -154.8997) -> (-0.08, -165.0997)
  line L621 (6.02, -190.1995) -> (6.02, -192.839)
  line L622 (1.72, -162.6997) -> (1.72, -157.2997)
  line L623 (18.12, -57.2997) -> (18.12, -62.6997)
  line L624 (-0.08, -54.8997) -> (-0.08, -65.0997)
  line L625 (13.82, -112.839) -> (13.82, -110.1995)
  line L626 (18.12, -157.2997) -> (18.12, -162.6997)
  line L627 (18.12, -157.2997) -> (18.12, -162.6997)
  line L628 (19.92, -65.0997) -> (19.92, -54.8997)
  line L629 (19.92, -165.0997) -> (19.92, -154.8997)
  line L630 (1.72, -162.6997) -> (1.72, -157.2997)
  line L631 (-0.08, -154.8997) -> (-0.08, -165.0997)
  line L632 (19.92, -165.0997) -> (19.92, -154.8997)
  circle A44 centre (9.92, -189.9997) radius 2.1
  line L633 (6.02, -190.1995) -> (6.02, -192.839)
  circle A45 centre (9.92, -189.9997) radius 2.1
  line L634 (1.72, -62.6997) -> (1.72, -57.2997)
  line L635 (13.82, -192.839) -> (13.82, -190.1995)
  line L636 (18.4614, -206.8782) -> (19.7422, -205.5975)
  line L637 (-0.08, -174.8997) -> (-0.08, -185.0997)
  line L638 (19.92, -85.1682) -> (19.92, -81.4997)
  line L639 (19.92, -85.1682) -> (19.92, -81.4997)
  arc A46 (1.3786, -206.8782) -> (1.72, -206.7368) centre (1.52, -206.7368) ccw
  arc A47 (1.72, -193.2625) -> (1.3786, -193.1211) centre (1.52, -193.2625) ccw
  line L640 (9.713, -106.0997) -> (7.0807, -106.0997)
  line L641 (-0.0748, -194.7519) -> (-0.0787, -194.7914)
  line L642 (12.7593, -173.8997) -> (16.1593, -177.2997)
  line L643 (18.4614, -26.8782) -> (19.7422, -25.5975)
  line L644 (-0.0593, -105.3253) -> (-0.0478, -105.3633)
  line L645 (0.0223, -105.5055) -> (0.0454, -105.5378)
  line L646 (13.82, -192.839) -> (13.82, -190.1995)
  line L647 (-0.08, -81.4997) -> (-0.08, -85.0997)
  line L648 (-0.08, -105.0997) -> (-0.0787, -105.2079)
  line L649 (0.0454, -105.5378) -> (0.0706, -105.5685)
  line L650 (-0.0683, -105.2866) -> (-0.0593, -105.3253)
  line L651 (15.42, -81.7997) -> (15.42, -83.439)
  arc A48 (1.3786, -106.8782) -> (1.72, -106.7368) centre (1.52, -106.7368) ccw
  line L652 (4.42, -83.439) -> (4.42, -81.7997)
  line L653 (3.6807, -177.2997) -> (7.0807, -173.8997)
  line L654 (-0.0338, -105.4005) -> (-0.0174, -105.4367)
  line L655 (-0.08, -105.0997) -> (-0.0787, -105.2079)
  line L656 (-0.08, -174.8997) -> (-0.08, -185.0997)
  line L657 (10.127, -106.0997) -> (9.92, -106.3066)
  line L658 (6.02, -109.7998) -> (6.2199, -109.9997)
  line L659 (0.0013, -105.4717) -> (0.0223, -105.5055)
  line L660 (18.12, -57.2997) -> (18.12, -62.6997)
  line L661 (12.7593, -173.8997) -> (16.1593, -177.2997)
  line L662 (19.92, -185.0997) -> (19.92, -174.8997)
  line L663 (3.3593, -204.4997) -> (6.02, -207.1603)
  line L664 (3.6807, -177.2997) -> (7.0807, -173.8997)
  line L665 (0.0223, -105.5055) -> (0.0454, -105.5378)
  line L666 (-0.08, -81.4997) -> (-0.08, -85.0997)
  line L667 (-0.0748, -105.2474) -> (-0.0683, -105.2866)
  line L668 (0.0454, -105.5378) -> (0.0706, -105.5685)
  line L669 (0.0978, -105.5975) -> (1.3786, -106.8782)
  line L670 (0.0706, -105.5685) -> (0.0978, -105.5975)
  line L671 (3.3593, -204.4997) -> (6.02, -207.1603)
  line L672 (4.42, -83.439) -> (4.42, -81.7997)
  line L673 (-0.0683, -105.2866) -> (-0.0593, -105.3253)
  line L674 (0.0978, -205.5975) -> (1.3786, -206.8782)
  arc A49 (18.12, -206.7368) -> (18.4614, -206.8782) centre (18.32, -206.7368) ccw
  line L675 (0.0013, -105.4717) -> (0.0223, -105.5055)
  line L676 (-0.0478, -105.3633) -> (-0.0338, -105.4005)
  line L677 (-0.0174, -105.4367) -> (0.0013, -105.4717)
  line L678 (-0.0338, -105.4005) -> (-0.0174, -105.4367)
  line L679 (-0.0593, -105.3253) -> (-0.0478, -105.3633)
  line L680 (1.72, -62.6997) -> (1.72, -57.2997)
  arc A50 (1.3786, -26.8782) -> (1.72, -26.7368) centre (1.52, -26.7368) ccw
  line L681 (-0.0787, -105.2079) -> (-0.0748, -105.2474)
  line L682 (0.0978, -105.5975) -> (1.3786, -106.8782)
  line L683 (15.42, -81.7997) -> (15.42, -83.439)
  line L684 (0.0706, -105.5685) -> (0.0978, -105.5975)
  line L685 (13.82, -27.1603) -> (16.4807, -24.4997)
  line L686 (-0.0748, -105.2474) -> (-0.0683, -105.2866)
  arc A51 (1.3786, -106.8782) -> (1.72, -106.7368) centre (1.52, -106.7368) ccw
  line L687 (-0.0478, -105.3633) -> (-0.0338, -105.4005)
  line L688 (-0.0787, -105.2079) -> (-0.0748, -105.2474)
  line L689 (19.92, -185.0997) -> (19.92, -174.8997)
  line L690 (-0.0174, -105.4367) -> (0.0013, -105.4717)
  line L691 (0.0978, -25.5975) -> (1.3786, -26.8782)
  line L692 (3.3593, -24.4997) -> (6.02, -27.1603)
  line L693 (0.0978, -194.4019) -> (0.0706, -194.4308)
  line L694 (3.6807, -182.6997) -> (1.72, -182.6997)
  line L695 (-0.0174, -194.5626) -> (-0.0338, -194.5988)
  line L696 (-0.0478, -54.636) -> (-0.0593, -54.674)
  line L697 (1.72, -177.2997) -> (3.6807, -177.2997)
  line L698 (0.0454, -54.4616) -> (0.0223, -54.4938)
  line L699 (1.72, -97.2997) -> (3.6807, -97.2997)
  line L700 (-0.0683, -54.7127) -> (-0.0748, -54.7519)
  line L701 (-0.0174, -54.5626) -> (-0.0338, -54.5988)
  line L702 (1.72, -55.4997) -> (1.72, -53.2625)
  line L703 (0.0706, -194.4308) -> (0.0454, -194.4616)
  line L704 (1.72, -182.6997) -> (1.72, -177.2997)
  line L705 (-0.0338, -54.5988) -> (-0.0478, -54.636)
  line L706 (-0.0478, -194.636) -> (-0.0593, -194.674)
  line L707 (0.0706, -54.4308) -> (0.0454, -54.4616)
  line L708 (10.127, -106.0997) -> (9.92, -106.3066)
  line L709 (0.0223, -194.4938) -> (0.0013, -194.5276)
  line L710 (9.713, -106.0997) -> (7.0807, -106.0997)
  line L711 (1.72, -195.4997) -> (1.72, -193.2625)
  line L712 (1.72, -182.6997) -> (1.72, -177.2997)
  line L713 (0.0454, -194.4616) -> (0.0223, -194.4938)
  line L714 (0.0454, -54.4616) -> (0.0223, -54.4938)
  line L715 (-0.0593, -54.674) -> (-0.0683, -54.7127)
  line L716 (-0.0478, -54.636) -> (-0.0593, -54.674)
  line L717 (1.72, -202.6997) -> (1.72, -197.2997)
  line L718 (6.2199, -109.9997) -> (6.02, -110.1995)
  arc A52 (1.72, -53.2625) -> (1.3786, -53.1211) centre (1.52, -53.2625) ccw
  line L719 (9.92, -106.3066) -> (9.713, -106.0997)
  line L720 (6.02, -109.7998) -> (6.2199, -109.9997)
  line L721 (6.02, -107.1603) -> (6.02, -109.7998)
  line L722 (3.6807, -182.6997) -> (1.72, -182.6997)
  line L723 (9.92, -106.3066) -> (9.713, -106.0997)
  line L724 (1.72, -184.4997) -> (3.3593, -184.4997)
  line L725 (6.2199, -109.9997) -> (6.02, -110.1995)
  line L726 (1.72, -195.4997) -> (1.72, -193.2625)
  line L727 (0.0978, -194.4019) -> (0.0706, -194.4308)
  line L728 (-0.0748, -54.7519) -> (-0.0787, -54.7914)
  line L729 (1.72, -104.4997) -> (3.3593, -104.4997)
  line L730 (0.0013, -194.5276) -> (-0.0174, -194.5626)
  line L731 (3.6807, -102.6997) -> (1.72, -102.6997)
  line L732 (-0.0683, -54.7127) -> (-0.0748, -54.7519)
  line L733 (-0.0683, -194.7127) -> (-0.0748, -194.7519)
  line L734 (1.72, -177.2997) -> (3.6807, -177.2997)
  line L735 (1.72, -104.4997) -> (3.3593, -104.4997)
  line L736 (3.6807, -102.6997) -> (1.72, -102.6997)
  line L737 (6.02, -107.1603) -> (6.02, -109.7998)
  line L738 (1.3786, -193.1211) -> (0.0978, -194.4019)
  line L739 (-0.0787, -54.7914) -> (-0.08, -54.8997)
  line L740 (0.0978, -54.4019) -> (0.0706, -54.4308)
  line L741 (-0.0787, -194.7914) -> (-0.08, -194.8997)
  line L742 (1.72, -97.2997) -> (3.6807, -97.2997)
  line L743 (1.72, -102.6997) -> (1.72, -97.2997)
  line L744 (7.0807, -106.0997) -> (3.6807, -102.6997)
  line L745 (0.0706, -54.4308) -> (0.0454, -54.4616)
  line L746 (1.3786, -193.1211) -> (0.0978, -194.4019)
  line L747 (1.72, -106.7368) -> (1.72, -104.4997)
  line L748 (0.0223, -54.4938) -> (0.0013, -54.5276)
  arc A53 (1.72, -193.2625) -> (1.3786, -193.1211) centre (1.52, -193.2625) ccw
  line L749 (1.72, -184.4997) -> (3.3593, -184.4997)
  line L750 (-0.0338, -194.5988) -> (-0.0478, -194.636)
  line L751 (1.72, -55.4997) -> (1.72, -53.2625)
  line L752 (1.72, -102.6997) -> (1.72, -97.2997)
  line L753 (1.72, -106.7368) -> (1.72, -104.4997)
  arc A54 (1.3786, -186.8782) -> (1.72, -186.7368) centre (1.52, -186.7368) ccw
  line L754 (-0.0787, -194.7914) -> (-0.08, -194.8997)
  line L755 (0.0454, -194.4616) -> (0.0223, -194.4938)
  line L756 (-0.0174, -54.5626) -> (-0.0338, -54.5988)
  line L757 (0.0013, -185.4717) -> (0.0223, -185.5055)
  line L758 (1.72, -206.7368) -> (1.72, -204.4997)
  line L759 (0.0223, -194.4938) -> (0.0013, -194.5276)
  line L760 (-0.08, -185.0997) -> (-0.0787, -185.2079)
  line L761 (1.3786, -53.1211) -> (0.0978, -54.4019)
  line L762 (0.0013, -194.5276) -> (-0.0174, -194.5626)
  line L763 (19.8738, -105.4005) -> (19.8878, -105.3633)
  line L764 (19.7946, -105.5378) -> (19.8177, -105.5055)
  line L765 (3.3593, -104.4997) -> (6.02, -107.1603)
  line L766 (-0.0478, -185.3633) -> (-0.0338, -185.4005)
  arc A55 (1.72, -53.2625) -> (1.3786, -53.1211) centre (1.52, -53.2625) ccw
  line L767 (0.0013, -54.5276) -> (-0.0174, -54.5626)
  line L768 (-0.0748, -54.7519) -> (-0.0787, -54.7914)
  line L769 (13.82, -110.1995) -> (13.6201, -109.9997)
  line L770 (0.0223, -185.5055) -> (0.0454, -185.5378)
  line L771 (1.3786, -53.1211) -> (0.0978, -54.4019)
  line L772 (-0.0593, -194.674) -> (-0.0683, -194.7127)
  line L773 (0.0706, -194.4308) -> (0.0454, -194.4616)
  line L774 (-0.0338, -54.5988) -> (-0.0478, -54.636)
  line L775 (13.6201, -109.9997) -> (13.82, -109.7998)
  line L776 (0.0454, -185.5378) -> (0.0706, -185.5685)
  line L777 (0.0223, -54.4938) -> (0.0013, -54.5276)
  line L778 (-0.0748, -185.2474) -> (-0.0683, -185.2866)
  line L779 (-0.0174, -185.4367) -> (0.0013, -185.4717)
  line L780 (-0.0593, -185.3253) -> (-0.0478, -185.3633)
  line L781 (-0.0748, -185.2474) -> (-0.0683, -185.2866)
  line L782 (-0.0593, -194.674) -> (-0.0683, -194.7127)
  line L783 (1.72, -202.6997) -> (1.72, -197.2997)
  line L784 (0.0013, -54.5276) -> (-0.0174, -54.5626)
  line L785 (7.0807, -106.0997) -> (3.6807, -102.6997)
  line L786 (-0.0338, -194.5988) -> (-0.0478, -194.636)
  line L787 (-0.0174, -194.5626) -> (-0.0338, -194.5988)
  line L788 (-0.0593, -54.674) -> (-0.0683, -54.7127)
  line L789 (-0.0338, -185.4005) -> (-0.0174, -185.4367)
  line L790 (3.3593, -104.4997) -> (6.02, -107.1603)
  line L791 (-0.0478, -194.636) -> (-0.0593, -194.674)
  line L792 (0.0978, -185.5975) -> (1.3786, -186.8782)
  line L793 (0.0454, -185.5378) -> (0.0706, -185.5685)
  arc A56 (18.12, -106.7368) -> (18.4614, -106.8782) centre (18.32, -106.7368) ccw
  line L794 (0.0978, -185.5975) -> (1.3786, -186.8782)
  line L795 (0.0223, -205.5055) -> (0.0454, -205.5378)
  line L796 (-0.0683, -194.7127) -> (-0.0748, -194.7519)
  line L797 (-0.0787, -45.2079) -> (-0.0748, -45.2474)
  line L798 (13.82, -110.1995) -> (13.6201, -109.9997)
  line L799 (0.0706, -185.5685) -> (0.0978, -185.5975)
  line L800 (-0.0683, -185.2866) -> (-0.0593, -185.3253)
  line L801 (-0.0683, -185.2866) -> (-0.0593, -185.3253)
  line L802 (-0.0174, -185.4367) -> (0.0013, -185.4717)
  line L803 (-0.0338, -185.4005) -> (-0.0174, -185.4367)
  line L804 (0.0978, -54.4019) -> (0.0706, -54.4308)
  arc A57 (1.3786, -186.8782) -> (1.72, -186.7368) centre (1.52, -186.7368) ccw
  line L805 (-0.0748, -194.7519) -> (-0.0787, -194.7914)
  line L806 (-0.0593, -205.3253) -> (-0.0478, -205.3633)
  line L807 (0.0013, -185.4717) -> (0.0223, -185.5055)
  line L808 (-0.0787, -54.7914) -> (-0.08, -54.8997)
  line L809 (-0.0593, -185.3253) -> (-0.0478, -185.3633)
  line L810 (0.0706, -185.5685) -> (0.0978, -185.5975)
  line L811 (13.6201, -109.9997) -> (13.82, -109.7998)
  line L812 (-0.0787, -185.2079) -> (-0.0748, -185.2474)
  line L813 (-0.0787, -185.2079) -> (-0.0748, -185.2474)
  line L814 (1.72, -46.7368) -> (1.72, -44.4997)
  line L815 (18.4614, -106.8782) -> (19.7422, -105.5975)
  line L816 (19.7694, -105.5685) -> (19.7946, -105.5378)
  line L817 (0.0454, -45.5378) -> (0.0706, -45.5685)
  line L818 (0.0706, -45.5685) -> (0.0978, -45.5975)
  line L819 (-0.08, -205.0997) -> (-0.0787, -205.2079)
  line L820 (19.8574, -105.4367) -> (19.8738, -105.4005)